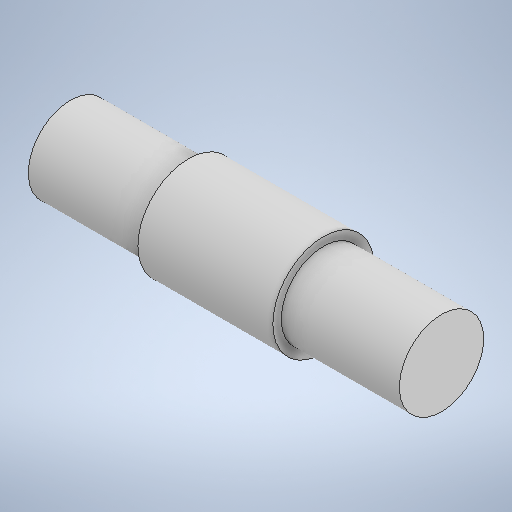
# Autodesk Inventor part: welle 6
Saved by Autodesk Inventor 2025.1 (Build 291241000, 241)
## iProperties
Created: 2024-09-13
Part Number: welle 6
Material: Generisch
Document SubType Name: Modeling
Designer: ffogue
Density: 1 g/cm^3
Appearance: Vorgabe
Author: ffogue
Autodesk Inventor part; units mm, degrees
ref_plane "YZ Plane" through (0, 0, 0) normal (1, 0, 0) x (0, 1, 0)
ref_plane "XZ Plane" through (0, 0, 0) normal (0, 1, 0) x (-1, 0, 0)
ref_plane "XY Plane" through (0, 0, 0) normal (0, 0, 1) x (1, 0, 0)
sketch "Sketch1" plane through (0, 0, 0) normal (0, 0, 1) x (1, 0, 0)
  line L0 (-11, 0) -> (-11, 2.5)
  line L1 (-11, 2.5) -> (-4, 2.5)
  line L2 (-4, 2.5) -> (-4, 3)
  line L3 (-4, 3) -> (4, 3)
  line L4 (4, 3) -> (4, 2.5)
  line L5 (4, 2.5) -> (11, 2.5)
  line L6 (11, 2.5) -> (11, 0)
  line L7 (11, 0) -> (-11, 0)
  point P0 (0, 0)
  point P1 (0, 0)
  dimension "d0" = 5
  dimension "d1" = 6
  dimension "d2" = 7
  dimension "d3" = 7
  dimension "d4" = 8
  constraints: 16 end point, 6 perpendicular, 2 point on line, 1 coincident, 1 midpoint, 1 vertical
  measures "d0" diameter of L1 L7
  measures "d1" diameter of L3 L7
  measures "d2" distance of L0.end L1.end
  measures "d3" distance of L4.end L5.end
  measures "d4" distance of L2.end L3.end
revolve "Revolution1" add sketch "Sketch1" angle 360 about axis through (11, 0, 0) along (-1, 0, 0)
body "Solid1"
